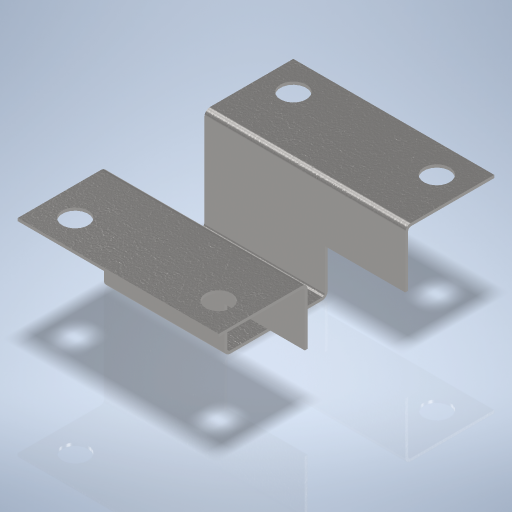
# Autodesk Inventor part: Bügelbefestigung
Saved by Autodesk Inventor 2024 (Build 280153000, 153)
## iProperties
Created: 2024-01-15
Part Number: Bügelbefestigung
Material: Stahl, galvanisiert
Document SubType Name: Sheet Metal
Designer: ffogue
Density: 7.85 g/cm^3
Sheet Metal Rule: Standard_mm
Appearance: Galvanisiert
Author: ffogue
Autodesk Inventor part; units mm, degrees
note: some values were not read from the file. Chosen so that the rebuilt part matches the saved one: direction of "Bohrung1".
ref_plane "YZ Plane" through (0, 0, 0) normal (1, 0, 0) x (0, 1, 0)
ref_plane "XZ Plane" through (0, 0, 0) normal (0, 1, 0) x (-1, 0, 0)
ref_plane "XY Plane" through (0, 0, 0) normal (0, 0, 1) x (1, 0, 0)
sketch "Skizze2" plane through (0, 0, 0) normal (0, 0, 1) x (1, 0, 0)
  line L0 (0, 18) -> (35, 18)
  line L1 (35, 18) -> (35, 0)
  line L2 (35, 0) -> (0, 0)
  line L3 (0, 0) -> (0, 18)
  dimension "d12" = 18
  dimension "d13" = 35
  measures "d12" distance between parallel lines of L2 L0
  measures "d13" distance of L1.end L2.end
extrude "Grobblech2" add sketch "Skizze2" along normal blind 0.5
sketch "Skizze3" plane through (0, 17.5, 0) normal (0, 1, 0) x (-1, 0, 0)
  line L0 (-35, 0) -> (0, 0)
  line L1 (0, 0) -> (0, 18)
  line L2 (0, 18) -> (-35, 18)
  line L3 (-35, 18) -> (-35, 0)
  constraints: 6 end point, 1 horizontal, 1 perpendicular, 1 vertical
edge flange "Lasche1" height 18 angle 90 thickness 0.5 bend radius 0.5 thickness toward (0, 1, 0) relief tear relief width 0.5 relief depth 0.25 edges at (17.5, 18, 0.5) wall of the first edge with corners at (35, 17.5, 0) (0, 17.5, 0) (0, 17.5, 18) (35, 17.5, 18)
bend "Biegung1"
corner "Ecke1"
sketch "Skizze4" plane through (35, 0.5, 0) normal (0, -1, 0) x (1, 0, 0)
  line L0 (-35, 0) -> (0, 0)
  line L1 (0, 0) -> (0, 18)
  line L2 (0, 18) -> (-35, 18)
  line L3 (-35, 18) -> (-35, 0)
  constraints: 6 end point, 1 horizontal, 1 perpendicular, 1 vertical
edge flange "Lasche2" height 18 angle 90 thickness 0.5 bend radius 0.5 thickness toward (0, -1, 0) relief tear relief width 0.5 relief depth 0.25 edges at (17.5, 0, 0.5) wall of the first edge with corners at (0, 0.5, 0) (35, 0.5, 0) (35, 0.5, 18) (0, 0.5, 18)
bend "Biegung2"
corner "Ecke2"
sketch "Skizze5" plane through (35, 17.5, 17.5) normal (0, 0, 1) x (1, 0, 0)
  line L0 (-35, 0) -> (0, 0)
  line L1 (0, 0) -> (0, 15.5)
  line L2 (0, 15.5) -> (-35, 15.5)
  line L3 (-35, 15.5) -> (-35, 0)
  constraints: 6 end point, 1 horizontal, 1 perpendicular, 1 vertical
edge flange "Lasche3" height 15.5 angle 90 thickness 0.5 bend radius 0.5 thickness toward (0, 0, 1) relief tear relief width 0.5 relief depth 0.25 edges at (17.5, 18, 18) wall of the first edge with corners at (0, 17.5, 17.5) (35, 17.5, 17.5) (35, 33, 17.5) (0, 33, 17.5)
bend "Biegung3"
corner "Ecke3"
sketch "Skizze6" plane through (0, 0.5, 17.5) normal (0, 0, 1) x (1, 0, 0)
  line L0 (35, 0) -> (0, 0)
  line L1 (0, 0) -> (0, -15.5)
  line L2 (0, -15.5) -> (35, -15.5)
  line L3 (35, -15.5) -> (35, 0)
  constraints: 6 end point, 1 horizontal, 1 perpendicular, 1 vertical
edge flange "Lasche4" height 15.5 angle 90 thickness 0.5 bend radius 0.5 thickness toward (0, 0, 1) relief tear relief width 0.5 relief depth 0.25 edges at (17.5, 0, 18) wall of the first edge with corners at (35, 0.5, 17.5) (0, 0.5, 17.5) (0, -15, 17.5) (35, -15, 17.5)
bend "Biegung4"
corner "Ecke4"
sketch "Skizze7" plane through (0, 0, 1) normal (0, -1, 0) x (1, 0, 0)
  line L0 (35, -1) -> (21, -1)
  line L1 (21, -1) -> (21, 7)
  line L2 (21, 7) -> (35, 7)
  line L3 (35, 7) -> (35, -1)
  line L4 (35, -1) -> (0, -1) projected
  dimension "d55" = 8
  dimension "d56" = 14
  constraints: 8 end point, 2 parallel, 1 horizontal, 1 perpendicular
  measures "d55" distance between parallel lines of L2 L0
  measures "d56" distance between parallel lines of L1 L3
extrude "Ausschneiden1" cut sketch "Skizze7" against normal up to surface (18 mm away)
sketch "Skizze8" plane through (0, 0, 0) normal (0, 0, -1) x (-1, 0, 0)
  line L0 (-21, 17) -> (-21, 1) projected
  line L1 (-21, 1) -> (0, 1) projected
  line L2 (0, 17) -> (0, 1) projected
  line L3 (0, 17) -> (-21, 17) projected
  line L4 (0, 9) -> (-30.5159, 9) construction
  line L5 (-35, -15) -> (0, -15) projected
  line L6 (-17.5, -15) -> (-17.5, 33) construction
  line L7 (0, 33) -> (-35, 33) projected
  point P0 (0, 0)
  point P1 (-30, 28)
  point P2 (-5, 28)
  point P3 (-30, -10)
  point P4 (-5, -10)
  dimension "d59" = 25
  dimension "d60" = 38
  dimension "d61" = 25
  dimension "d62" = 38
  constraints: 4 end point, 3 midpoint, 2 symmetric about line, 1 horizontal
  measures "d59" distance of point (-5, 28) point (-30, 28)
  measures "d60" distance of point (-5, 28) point (-5, -10)
  measures "d61" distance of point (-5, -10) point (-30, -10)
  measures "d62" distance of point (-30, 28) point (-30, -10)
hole "Bohrung1" at (30, 28, 0) at (5, 28, 0) at (30, -10, 0) at (5, -10, 0) direction (0, 0, 1) diameter 4.5 depth 18
sketch "Skizze9" plane through (0, 0, 0) normal (0, 0, -1) x (-1, 0, 0)
  line L0 (0, 17) -> (0, 1) projected
  point P0 (0, 0)
  point P1 (-8, 8.1851)
  point P2 (-16, 8.1851)
  dimension "d70" = 8
  dimension "d71" = 8
  measures "d70" distance of point (-8, 8.185) point (-16, 8.185)
  measures "d71" distance from line of L0 point (-8, 8.185)
hole "Bohrung2" at (8, 8.1851, 0) at (16, 8.1851, 0) direction (0, 0, 1) diameter 3 end through all
equation "\"d57\" = Stärke"
equation "\"d68\" = Stärke"
equation "\"d14\" = Stärke"
equation "\"d15\" = BreiteBiegungsfreistellung"
equation "\"d16\" = TiefeBiegungsfreistellung"
equation "\"d17\" = MinimalRest"
equation "\"d18\" = Übergangsradius"
equation "\"d21\" = Biegeradius"
equation "\"d22\" = GrößeEckenfreistellung"
equation "\"d23\" = Abstandsgröße"
equation "\"d24\" = JacobiRadiusGröße"
equation "\"d25\" = BreiteBiegungsfreistellung"
equation "\"d26\" = TiefeBiegungsfreistellung"
equation "\"d27\" = MinimalRest"
equation "\"d28\" = Übergangsradius"
equation "\"d31\" = Biegeradius"
equation "\"d32\" = GrößeEckenfreistellung"
equation "\"d33\" = Abstandsgröße"
equation "\"d34\" = JacobiRadiusGröße"
equation "\"d35\" = BreiteBiegungsfreistellung"
equation "\"d36\" = TiefeBiegungsfreistellung"
equation "\"d37\" = MinimalRest"
equation "\"d38\" = Übergangsradius"
equation "\"d41\" = Biegeradius"
equation "\"d42\" = GrößeEckenfreistellung"
equation "\"d43\" = Abstandsgröße"
equation "\"d44\" = JacobiRadiusGröße"
equation "\"d45\" = BreiteBiegungsfreistellung"
equation "\"d46\" = TiefeBiegungsfreistellung"
equation "\"d47\" = MinimalRest"
equation "\"d48\" = Übergangsradius"
equation "\"d51\" = Biegeradius"
equation "\"d52\" = GrößeEckenfreistellung"
equation "\"d53\" = Abstandsgröße"
equation "\"d54\" = JacobiRadiusGröße"
equation "\"Biegeradius\" = Stärke"
equation "\"BreiteBiegungsfreistellung\" = Stärke"
equation "\"TiefeBiegungsfreistellung\" = 0.5 * Stärke"
equation "\"GrößeEckenfreistellung\" = 4 * Stärke"
equation "\"MinimalRest\" = 2 * Stärke"
equation "\"Übergangsradius\" = Biegeradius"
equation "\"JacobiRadiusGröße\" = Biegeradius"
equation "\"Abstandsgröße\" = Stärke"
equation "\"Stärke\" = 0.5"
